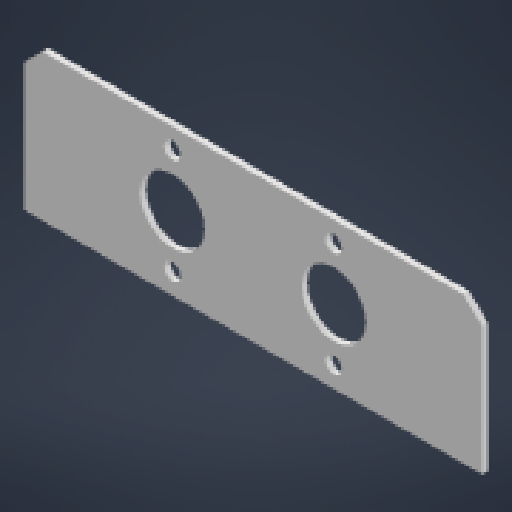
# Autodesk Inventor part: Pedalbox_V2_Vert_Rectangle
Saved by Autodesk Inventor 2027 (Build 310192000, 192)
## iProperties
Created: 2026-09-15
Part Number: Pedalbox_V2_Vert_Rectangle
Material: Generic
Document SubType Name: Modeling
Designer: share
Density: 1 g/cm^3
Appearance: Default
Author: share
Autodesk Inventor part; units mm, degrees
ref_plane "YZ Plane" through (0, 0, 0) normal (1, 0, 0) x (0, 1, 0)
ref_plane "XZ Plane" through (0, 0, 0) normal (0, 1, 0) x (-1, 0, 0)
ref_plane "XY Plane" through (0, 0, 0) normal (0, 0, 1) x (1, 0, 0)
sketch "Sketch1" plane through (0, 0, 0) normal (0, 0, 1) x (1, 0, 0)
  line L0 (125, -40) -> (-125, -40)
  line L1 (-125, -40) -> (-125, 40)
  line L2 (-125, 40) -> (125, 40)
  line L3 (125, 40) -> (125, -40)
  line L4 (0, 56) -> (0, -56) construction
  line L5 (-175, 0) -> (175, 0) construction
  point P0 (0, 0)
  dimension "d0" = 250
  dimension "d1" = 80
  constraints: 8 end point, 2 parallel, 1 horizontal, 1 perpendicular, 2 other
  measures "d0" distance between parallel lines of L3 L1
  measures "d1" distance between parallel lines of L0 L2
extrude "Extrusion1" add sketch "Sketch1" along normal mid plane 3.175
sketch "Sketch2" plane through (0, 0, 1.5875) normal (0, 0, 1) x (1, 0, 0)
  line L0 (0, 56) -> (0, -56) construction
  line L1 (-175, 0) -> (175, 0) construction
  line L2 (-125, -40) -> (125, -40) projected
  circle A0 centre (-40, 0) radius 17.5
  circle A1 centre (40, 0) radius 17.5
  line L3 (-40, -28.575) -> (-40, 28.575) construction
  circle A2 centre (-40, 28.575) radius 4.5
  circle A3 centre (-40, -28.575) radius 4.5
  circle A4 centre (40, -28.575) radius 4.5
  circle A5 centre (40, 28.575) radius 4.5
  point P0 (0, 0)
  dimension "d4" = 40
  dimension "d5" = 80
  dimension "d6" = 35
  dimension "d7" = 57.15
  dimension "d8" = 9
  constraints: 8 coincident, 6 centre point, 4 equal radius, 3 symmetric about line, 2 end point, 1 midpoint, 1 vertical
  measures "d4" distance from line of point (-40, 0) L2
  measures "d5" distance of point (40, 0) point (-40, 0)
  measures "d6" diameter of A0
  measures "d7" distance of L3.start L3.end
  measures "d8" diameter of A2
extrude "Extrusion2" cut sketch "Sketch2" against normal up to surface (3.175 mm away)
chamfer "Chamfer1" distance 10 angle 45 2 edges at (125, 40, 0) (-125, 40, 0)
sketch "Sketch3" plane through (0, 0, 1.5875) normal (0, 0, 1) x (1, 0, 0)
  line L0 (125, -40) -> (-125, -40) projected
  line L1 (-125, -40) -> (125, -40)
  line L2 (125, -40) -> (125, -38.024)
  line L3 (125, -38.024) -> (-125, -38.024)
  line L4 (-125, -38.024) -> (-125, -40)
  point P0 (0, 0)
  dimension "d14" = 1.976
  dimension "d15" = 250
  constraints: 8 end point, 2 parallel, 1 horizontal, 1 perpendicular
  measures "d14" distance of L1.end L2.end
  measures "d15" distance of L2.end L3.end
ref_plane "Work Plane1" through (-125, -40, -144.1323) normal (0, 0, -1) x (0, 1, 0)
extrude "Extrusion3" cut sketch "Sketch3" against normal up to surface (145.7198 mm away)
body "Solid1"
